Autodesk Fusion 360 part; units mm, degrees
note: some values were not read from the file. Set by a fixed rule: which sketch regions a step uses.
(part 3 of 7)
sketch "Sketch57" plane through (0, 116.2145, -31.1396) normal (0, 0.965926, -0.258819) x (-1, 0, 0)
  line L0 (-36.6, 185) -> (-48.311, 185)
  arc A0 (-49.911, 186.6) -> (-48.311, 185) centre (-48.311, 186.6) ccw
  line L1 (-49.911, 186.6) -> (-49.911, 195.348)
  arc A1 (-48.311, 196.948) -> (-49.911, 195.348) centre (-48.311, 195.348) ccw
  line L2 (-48.311, 196.948) -> (-36.6, 196.948)
  arc A2 (-35, 195.348) -> (-36.6, 196.948) centre (-36.6, 195.348) ccw
  line L3 (-35, 195.348) -> (-35, 186.6)
  arc A3 (-36.6, 185) -> (-35, 186.6) centre (-36.6, 186.6) ccw
  line L4 (-55, 195.348) -> (-55, 186.6)
  arc A4 (-56.6, 185) -> (-55, 186.6) centre (-56.6, 186.6) ccw
  line L5 (-56.6, 185) -> (-68.3957, 185)
  arc A5 (-69.9957, 186.6) -> (-68.3957, 185) centre (-68.3957, 186.6) ccw
  line L6 (-69.9957, 186.6) -> (-69.9957, 195.348)
  arc A6 (-68.3957, 196.948) -> (-69.9957, 195.348) centre (-68.3957, 195.348) ccw
  line L7 (-68.3957, 196.948) -> (-56.6, 196.948)
  arc A7 (-55, 195.348) -> (-56.6, 196.948) centre (-56.6, 195.348) ccw
  line L8 (-35, 204.6984) -> (-35, 201.6)
  arc A8 (-36.6, 200) -> (-35, 201.6) centre (-36.6, 201.6) ccw
  line L9 (-36.6, 200) -> (-48.311, 200)
  arc A9 (-49.911, 201.6) -> (-48.311, 200) centre (-48.311, 201.6) ccw
  line L10 (-49.911, 201.6) -> (-49.911, 204.6984)
  arc A10 (-48.311, 206.2984) -> (-49.911, 204.6984) centre (-48.311, 204.6984) ccw
  line L11 (-48.311, 206.2984) -> (-36.6, 206.2984)
  arc A11 (-35, 204.6984) -> (-36.6, 206.2984) centre (-36.6, 204.6984) ccw
  line L12 (-55, 204.5671) -> (-55, 201.6)
  arc A12 (-56.6, 200) -> (-55, 201.6) centre (-56.6, 201.6) ccw
  line L13 (-56.6, 200) -> (-68.7895, 200)
  arc A13 (-70.3895, 201.6) -> (-68.7895, 200) centre (-68.7895, 201.6) ccw
  line L14 (-70.3895, 201.6) -> (-70.3895, 204.5671)
  arc A14 (-68.7895, 206.1671) -> (-70.3895, 204.5671) centre (-68.7895, 204.5671) ccw
  line L15 (-68.7895, 206.1671) -> (-56.6, 206.1671)
  arc A15 (-55, 204.5671) -> (-56.6, 206.1671) centre (-56.6, 204.5671) ccw
  line L16 (25, 185) -> (0, 175)
  line L17 (0, 175) -> (0, 180.1897)
  line L18 (0, 180.1897) -> (25, 190.1897)
  line L19 (25, 190.1897) -> (25, 185)
  line L20 (-5, 190) -> (-5, 184.9041)
  line L21 (-5, 184.9041) -> (-30, 189.9041)
  line L22 (-30, 189.9041) -> (-30, 195)
  line L23 (-30, 195) -> (-5, 190)
  line L24 (-30, 150) -> (-30, 155)
  line L25 (-30, 155) -> (-5, 150)
  line L26 (-5, 150) -> (-5, 145)
  line L27 (-5, 145) -> (-30, 150)
  line L28 (-30, 160) -> (-30, 165.149)
  line L29 (-30, 165.149) -> (-5, 160.149)
  line L30 (-5, 160.149) -> (-5, 155)
  line L31 (-5, 155) -> (-30, 160)
  line L32 (-30, 200) -> (-30, 205)
  line L33 (-30, 205) -> (-5, 200)
  line L34 (-5, 200) -> (-5, 195)
  line L35 (-5, 195) -> (-30, 200)
  line L36 (25, 180.1705) -> (25, 175)
  line L37 (25, 175) -> (0, 165)
  line L38 (0, 165) -> (0, 170)
  line L39 (0, 170) -> (25, 180.1705)
  line L40 (25, 155) -> (0, 145)
  line L41 (0, 145) -> (0, 150)
  line L42 (0, 150) -> (25, 160)
  line L43 (25, 160) -> (25, 155)
  line L44 (25, 195) -> (0, 185)
  line L45 (0, 185) -> (0, 190)
  line L46 (0, 190) -> (25, 200)
  line L47 (25, 200) -> (25, 195)
  line L48 (-30, 180) -> (-30, 184.9041)
  line L49 (-30, 184.9041) -> (-5, 180)
  line L50 (-5, 180) -> (-5, 175)
  line L51 (-5, 175) -> (-30, 180)
  line L52 (-30, 170) -> (-30, 175)
  line L53 (-30, 175) -> (-5, 170)
  line L54 (-5, 170) -> (-5, 165)
  line L55 (-5, 165) -> (-30, 170)
  line L56 (25, 205) -> (0, 195)
  line L57 (0, 195) -> (0, 200)
  line L58 (0, 200) -> (25, 210)
  line L59 (25, 210) -> (25, 205)
  line L60 (25, 165) -> (0, 155)
  line L61 (0, 155) -> (0, 160)
  line L62 (0, 160) -> (25, 170)
  line L63 (25, 170) -> (25, 165)
  line L64 (-109.8689, 117.075) -> (-111.5449, 117.075)
  arc A16 (-116.5449, 122.075) -> (-111.5449, 117.075) centre (-111.5449, 122.075) ccw
  line L65 (-116.5449, 122.075) -> (-116.5449, 197.0502)
  arc A17 (-111.5449, 202.0502) -> (-116.5449, 197.0502) centre (-111.5449, 197.0502) ccw
  line L66 (-111.5449, 202.0502) -> (-109.8689, 202.0502)
  arc A18 (-104.8689, 197.0502) -> (-109.8689, 202.0502) centre (-109.8689, 197.0502) ccw
  line L67 (-104.8689, 197.0502) -> (-104.8689, 122.075)
  arc A19 (-109.8689, 117.075) -> (-104.8689, 122.075) centre (-109.8689, 122.075) ccw
  line L68 (-35, 125) -> (-35, 117.5)
  arc A20 (-37.5, 115) -> (-35, 117.5) centre (-37.5, 117.5) ccw
  line L69 (-37.5, 115) -> (-65, 115)
  arc A21 (-70, 120) -> (-65, 115) centre (-65, 120) ccw
  line L70 (-70, 120) -> (-70, 125)
  arc A22 (-65, 130) -> (-70, 125) centre (-65, 125) ccw
  line L71 (-65, 130) -> (-40, 130)
  arc A23 (-35, 125) -> (-40, 130) centre (-40, 125) ccw
  line L72 (-95.5983, 117.0948) -> (-95.6526, 117.0948)
  arc A24 (-100.6526, 122.0948) -> (-95.6526, 117.0948) centre (-95.6526, 122.0948) ccw
  line L73 (-100.6526, 122.0948) -> (-100.6526, 154.3733)
  line L74 (-100.6526, 154.3733) -> (-90.5983, 154.3733)
  line L75 (-90.5983, 154.3733) -> (-90.5983, 122.0948)
  arc A25 (-95.5983, 117.0948) -> (-90.5983, 122.0948) centre (-95.5983, 122.0948) ccw
  arc A26 (-90.5983, 197.0502) -> (-95.5983, 202.0502) centre (-95.5983, 197.0502) ccw
  line L76 (-90.5983, 197.0502) -> (-90.5983, 159.5626)
  line L77 (-90.5983, 159.5626) -> (-100.6526, 159.5626)
  line L78 (-100.6526, 159.5626) -> (-100.6526, 197.0502)
  arc A27 (-95.6526, 202.0502) -> (-100.6526, 197.0502) centre (-95.6526, 197.0502) ccw
  line L79 (-95.6526, 202.0502) -> (-95.5983, 202.0502)
  line L80 (-37.5, 135) -> (-67.5, 135)
  arc A28 (-70, 137.5) -> (-67.5, 135) centre (-67.5, 137.5) ccw
  line L81 (-70, 137.5) -> (-70, 142.5)
  arc A29 (-67.5, 145) -> (-70, 142.5) centre (-67.5, 142.5) ccw
  line L82 (-67.5, 145) -> (-37.5, 145)
  arc A30 (-35, 142.5) -> (-37.5, 145) centre (-37.5, 142.5) ccw
  line L83 (-35, 142.5) -> (-35, 137.5)
  arc A31 (-37.5, 135) -> (-35, 137.5) centre (-37.5, 137.5) ccw
  arc A32 (-84.2974, 121.8844) -> (-80.3534, 116.9972) centre (-79.2974, 121.8844) ccw
  line L84 (-84.2974, 121.8844) -> (-84.2974, 171.0352)
  line L85 (-84.2974, 171.0352) -> (-76.4093, 171.0352)
  line L86 (-76.4093, 171.0352) -> (-76.4093, 121.8844)
  arc A33 (-80.3534, 116.9972) -> (-76.4093, 121.8844) centre (-81.4093, 121.8844) ccw
  arc A34 (-76.4093, 196.948) -> (-80.3534, 201.8353) centre (-81.4093, 196.948) ccw
  line L87 (-76.4093, 196.948) -> (-76.4093, 176.5782)
  line L88 (-76.4093, 176.5782) -> (-84.2974, 176.5782)
  line L89 (-84.2974, 176.5782) -> (-84.2974, 196.948)
  arc A35 (-80.3534, 201.8353) -> (-84.2974, 196.948) centre (-79.2974, 196.948) ccw
  line L90 (-120, 85) -> (-120, 100)
  arc A36 (-110, 110) -> (-120, 100) centre (-110, 100) ccw
  line L91 (-110, 110) -> (-61.6636, 110)
  arc A37 (-51.6636, 100) -> (-61.6636, 110) centre (-61.6636, 100) ccw
  line L92 (-51.6636, 100) -> (-51.6636, 85)
  arc A38 (-61.6636, 75) -> (-51.6636, 85) centre (-61.6636, 85) ccw
  line L93 (-61.6636, 75) -> (-110, 75)
  arc A39 (-120, 85) -> (-110, 75) centre (-110, 85) ccw
  line L94 (-45.44, 85) -> (-45.44, 100)
  arc A40 (-35.44, 110) -> (-45.44, 100) centre (-35.44, 100) ccw
  line L95 (-35.44, 110) -> (-20, 110)
  arc A41 (-10, 100) -> (-20, 110) centre (-20, 100) ccw
  line L96 (-10, 100) -> (-10, 85)
  arc A42 (-20, 75) -> (-10, 85) centre (-20, 85) ccw
  line L97 (-20, 75) -> (-35.44, 75)
  arc A43 (-45.44, 85) -> (-35.44, 75) centre (-35.44, 85) ccw
  line L98 (22.9316, 100) -> (22.9316, 85)
  arc A44 (12.9316, 75) -> (22.9316, 85) centre (12.9316, 85) ccw
  line L99 (12.9316, 75) -> (7.9281, 75)
  arc A45 (-2.0719, 85) -> (7.9281, 75) centre (7.9281, 85) ccw
  line L100 (-2.0719, 85) -> (-2.0719, 100)
  arc A46 (7.9281, 110) -> (-2.0719, 100) centre (7.9281, 100) ccw
  line L101 (7.9281, 110) -> (12.9316, 110)
  arc A47 (22.9316, 100) -> (12.9316, 110) centre (12.9316, 100) ccw
  line L102 (-40, 30) -> (-110, 30)
  arc A48 (-120, 40) -> (-110, 30) centre (-110, 40) ccw
  line L103 (-120, 40) -> (-120, 60)
  arc A49 (-110, 70) -> (-120, 60) centre (-110, 60) ccw
  line L104 (-110, 70) -> (-40, 70)
  arc A50 (-30, 60) -> (-40, 70) centre (-40, 60) ccw
  line L105 (-30, 60) -> (-30, 40)
  arc A51 (-40, 30) -> (-30, 40) centre (-40, 40) ccw
  line L106 (-10, 70) -> (10, 70)
  arc A52 (20, 60) -> (10, 70) centre (10, 60) ccw
  line L107 (20, 60) -> (20, 40)
  arc A53 (10, 30) -> (20, 40) centre (10, 40) ccw
  line L108 (10, 30) -> (-10, 30)
  arc A54 (-20, 40) -> (-10, 30) centre (-10, 40) ccw
  line L109 (-20, 40) -> (-20, 60)
  arc A55 (-10, 70) -> (-20, 60) centre (-10, 60) ccw
  ellipse E0 centre (22.741, -39.3535) end of major axis (22.741, -46.5838) minor radius 7 (22.741, -46.5838) -> (29.741, -39.3535) ccw
  line L110 (29.741, -39.3535) -> (29.741, 209.5755)
  ellipse E1 centre (22.741, 209.5755) end of major axis (22.741, 216.8058) minor radius 7 (29.741, 209.5755) -> (22.741, 216.8058) ccw
  line L111 (22.741, 216.8058) -> (-123.259, 216.8058)
  ellipse E2 centre (-123.259, 209.5755) end of major axis (-123.259, 216.8058) minor radius 7 (-123.259, 216.8058) -> (-130.259, 209.5755) ccw
  line L112 (-130.259, 209.5755) -> (-130.259, -39.3535)
  ellipse E3 centre (-123.259, -39.3535) end of major axis (-123.259, -46.5838) minor radius 7 (-130.259, -39.3535) -> (-123.259, -46.5838) ccw
  line L113 (-123.259, -46.5838) -> (22.741, -46.5838)
  line L114 (-35.9419, 179.9959) -> (-35.9419, 150.9959)
  line L115 (-35.9419, 150.9959) -> (-72.9419, 150.9959)
  line L116 (-72.9419, 150.9959) -> (-72.9419, 179.9959)
  line L117 (-72.9419, 179.9959) -> (-35.9419, 179.9959)
  circle A56 centre (-57, 13) radius 1.5
  dimension "d224" = 3
  measures "d224" diameter of A56
sketch "Sketch58" plane through (0, 0, 0) normal (0, 1, 0) x (1, 0, 0)
sketch "Sketch1 (2)" plane through (0, 0, 0) normal (0, 1, 0) x (1, 0, 0) in component "axe"
  line L0 (-180, -19.5879) -> (-227.1834, -19.5879)
  line L1 (-227.1834, -19.5879) -> (-227.1834, -2.995)
  line L2 (-227.1834, -2.995) -> (-170, -2.995)
  line L3 (-170, -2.995) -> (-170, -9.5879)
  line L4 (-189.6546, -2.995) -> (-208.419, -2.995)
  line L5 (-208.419, -2.995) -> (-208.419, 108.2304)
  line L6 (-208.419, 108.2304) -> (-189.6546, 108.2304)
  line L7 (-189.6546, 108.2304) -> (-189.6546, -2.995)
  arc A0 (-180, -19.5879) -> (-170, -9.5879) centre (-180, -9.5879) ccw
  dimension "d328" = 10
  dimension "d329" = 127.8184
  constraint horizontal L0
  constraint vertical L1
  constraint horizontal L2
  constraint vertical L3
  constraint horizontal L4
  constraint vertical L5
  constraint horizontal L6
  constraint vertical L7
  constraint coincident L2 L4.start
  constraint tangent L0 A0
  constraint tangent L3 A0
  measures "d328" radius of A0
  measures "d329" distance of L0 L6
extrude "Extrude1" add sketch "Sketch1 (2)" along normal blind 10 in component "axe"
shell "Shell1" thickness 1 removed faces 1 at (-202.1642, 3.3333, -108.2304) in component "axe"
move_body "Move1" bodies 1 to x (1, 0, 0) y (0, -1, 0) z (0, 0, -1) at (237.3583, 174.6092, -54.5958) in component "axe"
move_body "Move2" bodies 1 to x (0, 1, 0) y (-1, 0, 0) z (0, 0, 1) at (222.3129, 121.9056, 15) in component "axe"
move_body "Move3" bodies 1 to x (1, 0, 0) y (0, 0.258819, 0.965926) z (0, -0.965926, 0.258819) at (3.5, 142.9141, -113.2543) in component "axe"
move_body "Move4" bodies 1 to x (1, 0, 0) y (0, 1, 0) z (0, 0, 1) at (170, 47.007, -22.6429) in component "axe"
sketch "Sketch60" plane through (-29.741, 0, 0) normal (-1, 0, 0) x (0, 0, 1)
  line L0 (4.8558, 108) -> (45, 108)
  line L1 (45, 108) -> (45, 101.218)
  line L2 (45, 101.218) -> (4.8558, 101.218)
  line L3 (4.8558, 101.218) -> (4.8558, 108)
  line L4 (-69.1521, 106.0291) -> (-69.1009, 100.1665)
  line L5 (-69.1009, 100.1665) -> (171.8899, 102.2696)
  line L6 (171.8899, 102.2696) -> (171.2948, 170.4566)
  line L7 (171.2948, 170.4566) -> (-69.1521, 106.0291)
  line L8 (103.7389, 125) -> (70, 125)
  line L9 (65, 120) -> (65, 115.8193)
  line L10 (70, 110.8193) -> (103.7389, 110.8193)
  line L11 (108.7389, 115.8193) -> (108.7389, 120)
  arc A0 (70, 125) -> (65, 120) centre (70, 120) ccw
  arc A1 (65, 115.8193) -> (70, 110.8193) centre (70, 115.8193) ccw
  arc A2 (108.7389, 120) -> (103.7389, 125) centre (103.7389, 120) ccw
  arc A3 (103.7389, 110.8193) -> (108.7389, 115.8193) centre (103.7389, 115.8193) ccw
  dimension "d243" = 5
  dimension "d244" = 5
  constraint horizontal L8
  constraint vertical L9
  constraint horizontal L10
  constraint vertical L11
  constraint tangent L8 A0
  constraint tangent L9 A0
  constraint tangent L9 A1
  constraint tangent L10 A1
  constraint equal A0 A1
  constraint tangent L8 A2
  constraint tangent L11 A2
  constraint tangent L10 A3
  constraint tangent L11 A3
  constraint equal A2 A3
  measures "d243" radius of A0
  measures "d244" radius of A2
sketch "Sketch61" plane through (130.259, 0, 0) normal (1, 0, 0) x (0, 0, -1)
  line L0 (-45, 101.218) -> (-45, 110)
  line L1 (-45, 110) -> (-6.7003, 110)
  line L2 (-6.7003, 110) -> (-6.7003, 101.218)
  line L3 (-6.7003, 101.218) -> (-45, 101.218)
  line L4 (69.1009, 100.1665) -> (69.1521, 106.0291)
  line L5 (69.1521, 106.0291) -> (-171.2948, 170.4566)
  line L6 (-171.2948, 170.4566) -> (-171.8899, 102.2696)
  line L7 (-171.8899, 102.2696) -> (69.1009, 100.1665)
  line L8 (-108.8645, 127.2667) -> (-70.0825, 127.2667)
  line L9 (-66.3825, 123.5667) -> (-66.3825, 116.3937)
  line L10 (-70.0825, 112.6937) -> (-108.8645, 112.6937)
  line L11 (-112.5645, 116.3937) -> (-112.5645, 123.5667)
  arc A0 (-66.3825, 123.5667) -> (-70.0825, 127.2667) centre (-70.0825, 123.5667) ccw
  arc A1 (-70.0825, 112.6937) -> (-66.3825, 116.3937) centre (-70.0825, 116.3937) ccw
  arc A2 (-112.5645, 116.3937) -> (-108.8645, 112.6937) centre (-108.8645, 116.3937) ccw
  arc A3 (-108.8645, 127.2667) -> (-112.5645, 123.5667) centre (-108.8645, 123.5667) ccw
  dimension "d247" = 3.7
  constraint horizontal L8
  constraint horizontal L10
  constraint vertical L11
  constraint tangent L8 A0
  constraint tangent L9 A0
  constraint tangent L9 A1
  constraint tangent L10 A1
  constraint equal A0 A1
  constraint tangent L10 A2
  constraint tangent L11 A2
  constraint equal A0 A2
  constraint tangent L8 A3
  constraint tangent L11 A3
  constraint equal A0 A3
  measures "d247" radius of A0
sketch "Sketch62" plane through (-26.741, 0, 0) normal (1, 0, 0) x (0, 0, -1)
  line L0 (-175.8897, 102.3045) -> (73.1008, 100.1316)
  line L1 (73.1008, 100.1316) -> (73.1159, 101.8612)
  line L2 (73.1159, 101.8612) -> (-175.3127, 168.4274)
  line L3 (-175.3127, 168.4274) -> (-175.8897, 102.3045)
  line L4 (-101.4003, 140.9215) -> (-77.5652, 140.9215)
  line L5 (-77.5652, 140.9215) -> (-77.5652, 128.7199)
  line L6 (-77.5652, 128.7199) -> (-101.4003, 128.7199)
  line L7 (-101.4003, 128.7199) -> (-101.4003, 140.9215)
  constraint horizontal L4
  constraint vertical L5
  constraint horizontal L6
  constraint vertical L7
move_body "Move5" bodies 1 to x (1, 0, 0) y (0, 1, 0) z (0, 0, 1) at (-87, -50.9421, 56.6747) in component "axe"
sketch "Sketch64" plane through (0, 115.0071, -30.8161) normal (0, 0.965926, -0.258819) x (-1, 0, 0)
  arc A0 (-110, 110) -> (-120, 100) centre (-110, 100) ccw
  line L0 (-120, 100) -> (-120, 85)
  arc A1 (-120, 85) -> (-110, 75) centre (-110, 85) ccw
  line L1 (-110, 75) -> (-61.6636, 75)
  arc A2 (-61.6636, 75) -> (-51.6636, 85) centre (-61.6636, 85) ccw
  line L2 (-51.6636, 85) -> (-51.6636, 100)
  arc A3 (-51.6636, 100) -> (-61.6636, 110) centre (-61.6636, 100) ccw
  line L3 (-61.6636, 110) -> (-110, 110)
sketch "Sketch65" plane through (0, 115.0071, -30.8161) normal (0, 0.965926, -0.258819) x (-1, 0, 0)
  line L0 (-110, 110) -> (-82.9094, 110)
  line L1 (-82.9094, 110) -> (-82.9094, 88.2587)
  line L2 (-82.9094, 88.2587) -> (-110, 88.2587)
  line L3 (-110, 88.2587) -> (-110, 110)
  line L4 (-65, 80) -> (-96.4547, 80)
  line L5 (-96.4547, 80) -> (-96.4547, 101.0146)
  line L6 (-96.4547, 101.0146) -> (-65, 101.0146)
  line L7 (-65, 101.0146) -> (-65, 80)
  line L8 (-52.1358, 86.6643) -> (-76.8504, 86.6643)
  line L9 (-76.8504, 86.6643) -> (-76.8504, 104.6819)
  line L10 (-76.8504, 104.6819) -> (-52.1358, 104.6819)
  line L11 (-52.1358, 104.6819) -> (-52.1358, 86.6643)
  line L12 (-102.5797, 95.6731) -> (-115, 95.6731)
  line L13 (-115, 95.6731) -> (-115, 80)
  line L14 (-115, 80) -> (-102.5797, 80)
  line L15 (-102.5797, 80) -> (-102.5797, 95.6731)
  constraint horizontal L0
  constraint vertical L1
  constraint horizontal L2
  constraint vertical L3
  constraint horizontal L4
  constraint vertical L5
  constraint horizontal L6
  constraint vertical L7
  constraint horizontal L8
  constraint vertical L9
  constraint horizontal L10
  constraint vertical L11
  constraint horizontal L12
  constraint vertical L13
  constraint horizontal L14
  constraint vertical L15
sketch "Sketch66" plane through (0, 115.0071, -30.8161) normal (0, 0.965926, -0.258819) x (-1, 0, 0)
  line L0 (-110, 75) -> (-90, 75)
  line L1 (-90, 75) -> (-90, 95)
  line L2 (-90, 95) -> (-110, 95)
  line L3 (-110, 95) -> (-110, 75)
  line L4 (-60, 80) -> (-81.2122, 80)
  line L5 (-81.2122, 80) -> (-81.2122, 98.5014)
  line L6 (-81.2122, 98.5014) -> (-60, 98.5014)
  line L7 (-60, 98.5014) -> (-60, 80)
  constraint horizontal L0
  constraint vertical L1
  constraint horizontal L2
  constraint vertical L3
  constraint horizontal L4
  constraint vertical L5
  constraint horizontal L6
  constraint vertical L7
sketch "Sketch67" plane through (0, 115.973, -31.0749) normal (0, 0.965926, -0.258819) x (-1, 0, 0)
  line L0 (-60, 98.5014) -> (-81.2122, 98.5014)
  line L1 (-81.2122, 98.5014) -> (-81.2122, 80)
  line L2 (-81.2122, 80) -> (-60, 80)
  line L3 (-60, 80) -> (-60, 98.5014)
  circle A0 centre (-63, 96) radius 1.5
  circle A1 centre (-78, 96) radius 1.5
  circle A2 centre (-93, 92) radius 1.5
  circle A3 centre (-107, 92) radius 1.5
  dimension "d262" = 3
  dimension "d263" = 3
  dimension "d264" = 3
  dimension "d265" = 3
  measures "d262" diameter of A0
  measures "d263" diameter of A1
  measures "d264" diameter of A2
  measures "d265" diameter of A3
move_body "Move6" bodies 1 to x (1, 0, 0) y (0, 1, 0) z (0, 0, 1) at (138.1861, 0.7755, 2.894) in component "axe"
sketch "Sketch70" plane through (0, 116.2145, -31.1396) normal (0, 0.965926, -0.258819) x (-1, 0, 0)
  line L0 (-36.6, 185) -> (-48.311, 185)
  arc A0 (-49.911, 186.6) -> (-48.311, 185) centre (-48.311, 186.6) ccw
  line L1 (-49.911, 186.6) -> (-49.911, 195.348)
  arc A1 (-48.311, 196.948) -> (-49.911, 195.348) centre (-48.311, 195.348) ccw
  line L2 (-48.311, 196.948) -> (-36.6, 196.948)
  arc A2 (-35, 195.348) -> (-36.6, 196.948) centre (-36.6, 195.348) ccw
  line L3 (-35, 195.348) -> (-35, 186.6)
  arc A3 (-36.6, 185) -> (-35, 186.6) centre (-36.6, 186.6) ccw
  line L4 (-55, 195.348) -> (-55, 186.6)
  arc A4 (-56.6, 185) -> (-55, 186.6) centre (-56.6, 186.6) ccw
  line L5 (-56.6, 185) -> (-68.3957, 185)
  arc A5 (-69.9957, 186.6) -> (-68.3957, 185) centre (-68.3957, 186.6) ccw
  line L6 (-69.9957, 186.6) -> (-69.9957, 195.348)
  arc A6 (-68.3957, 196.948) -> (-69.9957, 195.348) centre (-68.3957, 195.348) ccw
  line L7 (-68.3957, 196.948) -> (-56.6, 196.948)
  arc A7 (-55, 195.348) -> (-56.6, 196.948) centre (-56.6, 195.348) ccw
  line L8 (-35, 204.6984) -> (-35, 201.6)
  arc A8 (-36.6, 200) -> (-35, 201.6) centre (-36.6, 201.6) ccw
  line L9 (-36.6, 200) -> (-48.311, 200)
  arc A9 (-49.911, 201.6) -> (-48.311, 200) centre (-48.311, 201.6) ccw
  line L10 (-49.911, 201.6) -> (-49.911, 204.6984)
  arc A10 (-48.311, 206.2984) -> (-49.911, 204.6984) centre (-48.311, 204.6984) ccw
  line L11 (-48.311, 206.2984) -> (-36.6, 206.2984)
  arc A11 (-35, 204.6984) -> (-36.6, 206.2984) centre (-36.6, 204.6984) ccw
  line L12 (-55, 204.5671) -> (-55, 201.6)
  arc A12 (-56.6, 200) -> (-55, 201.6) centre (-56.6, 201.6) ccw
  line L13 (-56.6, 200) -> (-68.7895, 200)
  arc A13 (-70.3895, 201.6) -> (-68.7895, 200) centre (-68.7895, 201.6) ccw
  line L14 (-70.3895, 201.6) -> (-70.3895, 204.5671)
  arc A14 (-68.7895, 206.1671) -> (-70.3895, 204.5671) centre (-68.7895, 204.5671) ccw
  line L15 (-68.7895, 206.1671) -> (-56.6, 206.1671)
  arc A15 (-55, 204.5671) -> (-56.6, 206.1671) centre (-56.6, 204.5671) ccw
  line L16 (25, 185) -> (0, 175)
  line L17 (0, 175) -> (0, 180.1897)
  line L18 (0, 180.1897) -> (25, 190.1897)
  line L19 (25, 190.1897) -> (25, 185)
  line L20 (-5, 190) -> (-5, 184.9041)
  line L21 (-5, 184.9041) -> (-30, 189.9041)
  line L22 (-30, 189.9041) -> (-30, 195)
  line L23 (-30, 195) -> (-5, 190)
  line L24 (-30, 150) -> (-30, 155)
  line L25 (-30, 155) -> (-5, 150)
  line L26 (-5, 150) -> (-5, 145)
  line L27 (-5, 145) -> (-30, 150)
  line L28 (-30, 160) -> (-30, 165.149)
  line L29 (-30, 165.149) -> (-5, 160.149)
  line L30 (-5, 160.149) -> (-5, 155)
  line L31 (-5, 155) -> (-30, 160)
  line L32 (-30, 200) -> (-30, 205)
  line L33 (-30, 205) -> (-5, 200)
  line L34 (-5, 200) -> (-5, 195)
  line L35 (-5, 195) -> (-30, 200)
  line L36 (25, 180.1705) -> (25, 175)
  line L37 (25, 175) -> (0, 165)
  line L38 (0, 165) -> (0, 170)
  line L39 (0, 170) -> (25, 180.1705)
  line L40 (25, 155) -> (0, 145)
  line L41 (0, 145) -> (0, 150)
  line L42 (0, 150) -> (25, 160)
  line L43 (25, 160) -> (25, 155)
  line L44 (25, 195) -> (0, 185)
  line L45 (0, 185) -> (0, 190)
  line L46 (0, 190) -> (25, 200)
  line L47 (25, 200) -> (25, 195)
  line L48 (-30, 180) -> (-30, 184.9041)
  line L49 (-30, 184.9041) -> (-5, 180)
  line L50 (-5, 180) -> (-5, 175)
  line L51 (-5, 175) -> (-30, 180)
  line L52 (-30, 170) -> (-30, 175)
  line L53 (-30, 175) -> (-5, 170)
  line L54 (-5, 170) -> (-5, 165)
  line L55 (-5, 165) -> (-30, 170)
  line L56 (25, 205) -> (0, 195)
  line L57 (0, 195) -> (0, 200)
  line L58 (0, 200) -> (25, 210)
  line L59 (25, 210) -> (25, 205)
  line L60 (25, 165) -> (0, 155)
  line L61 (0, 155) -> (0, 160)
  line L62 (0, 160) -> (25, 170)
  line L63 (25, 170) -> (25, 165)
  line L64 (-109.8689, 117.075) -> (-111.5449, 117.075)
  arc A16 (-116.5449, 122.075) -> (-111.5449, 117.075) centre (-111.5449, 122.075) ccw
  line L65 (-116.5449, 122.075) -> (-116.5449, 197.0502)
  arc A17 (-111.5449, 202.0502) -> (-116.5449, 197.0502) centre (-111.5449, 197.0502) ccw
  line L66 (-111.5449, 202.0502) -> (-109.8689, 202.0502)
  arc A18 (-104.8689, 197.0502) -> (-109.8689, 202.0502) centre (-109.8689, 197.0502) ccw
  line L67 (-104.8689, 197.0502) -> (-104.8689, 122.075)
  arc A19 (-109.8689, 117.075) -> (-104.8689, 122.075) centre (-109.8689, 122.075) ccw
  line L68 (-35, 125) -> (-35, 117.5)
  arc A20 (-37.5, 115) -> (-35, 117.5) centre (-37.5, 117.5) ccw
  line L69 (-37.5, 115) -> (-65, 115)
  arc A21 (-70, 120) -> (-65, 115) centre (-65, 120) ccw
  line L70 (-70, 120) -> (-70, 125)
  arc A22 (-65, 130) -> (-70, 125) centre (-65, 125) ccw
  line L71 (-65, 130) -> (-40, 130)
  arc A23 (-35, 125) -> (-40, 130) centre (-40, 125) ccw
  line L72 (-95.5983, 117.0948) -> (-95.6526, 117.0948)
  arc A24 (-100.6526, 122.0948) -> (-95.6526, 117.0948) centre (-95.6526, 122.0948) ccw
  line L73 (-100.6526, 122.0948) -> (-100.6526, 154.3733)
  line L74 (-100.6526, 154.3733) -> (-90.5983, 154.3733)
  line L75 (-90.5983, 154.3733) -> (-90.5983, 122.0948)
  arc A25 (-95.5983, 117.0948) -> (-90.5983, 122.0948) centre (-95.5983, 122.0948) ccw
  arc A26 (-90.5983, 197.0502) -> (-95.5983, 202.0502) centre (-95.5983, 197.0502) ccw
  line L76 (-90.5983, 197.0502) -> (-90.5983, 159.5626)
  line L77 (-90.5983, 159.5626) -> (-100.6526, 159.5626)
  line L78 (-100.6526, 159.5626) -> (-100.6526, 197.0502)
  arc A27 (-95.6526, 202.0502) -> (-100.6526, 197.0502) centre (-95.6526, 197.0502) ccw
  line L79 (-95.6526, 202.0502) -> (-95.5983, 202.0502)
  line L80 (-37.5, 135) -> (-67.5, 135)
  arc A28 (-70, 137.5) -> (-67.5, 135) centre (-67.5, 137.5) ccw
  line L81 (-70, 137.5) -> (-70, 142.5)
  arc A29 (-67.5, 145) -> (-70, 142.5) centre (-67.5, 142.5) ccw
  line L82 (-67.5, 145) -> (-37.5, 145)
  arc A30 (-35, 142.5) -> (-37.5, 145) centre (-37.5, 142.5) ccw
  line L83 (-35, 142.5) -> (-35, 137.5)
  arc A31 (-37.5, 135) -> (-35, 137.5) centre (-37.5, 137.5) ccw
  arc A32 (-84.2974, 121.8844) -> (-80.3534, 116.9972) centre (-79.2974, 121.8844) ccw
  line L84 (-84.2974, 121.8844) -> (-84.2974, 171.0352)
  line L85 (-84.2974, 171.0352) -> (-76.4093, 171.0352)
  line L86 (-76.4093, 171.0352) -> (-76.4093, 121.8844)
  arc A33 (-80.3534, 116.9972) -> (-76.4093, 121.8844) centre (-81.4093, 121.8844) ccw
  arc A34 (-76.4093, 196.948) -> (-80.3534, 201.8353) centre (-81.4093, 196.948) ccw
  line L87 (-76.4093, 196.948) -> (-76.4093, 176.5782)
  line L88 (-76.4093, 176.5782) -> (-84.2974, 176.5782)
  line L89 (-84.2974, 176.5782) -> (-84.2974, 196.948)
  arc A35 (-80.3534, 201.8353) -> (-84.2974, 196.948) centre (-79.2974, 196.948) ccw
  line L90 (-120, 85) -> (-120, 100)
  arc A36 (-110, 110) -> (-120, 100) centre (-110, 100) ccw
  line L91 (-110, 110) -> (-61.6636, 110)
  arc A37 (-51.6636, 100) -> (-61.6636, 110) centre (-61.6636, 100) ccw
  line L92 (-51.6636, 100) -> (-51.6636, 85)
  arc A38 (-61.6636, 75) -> (-51.6636, 85) centre (-61.6636, 85) ccw
  line L93 (-61.6636, 75) -> (-110, 75)
  arc A39 (-120, 85) -> (-110, 75) centre (-110, 85) ccw
  line L94 (-45.44, 85) -> (-45.44, 100)
  arc A40 (-35.44, 110) -> (-45.44, 100) centre (-35.44, 100) ccw
  line L95 (-35.44, 110) -> (-20, 110)
  arc A41 (-10, 100) -> (-20, 110) centre (-20, 100) ccw
  line L96 (-10, 100) -> (-10, 85)
  arc A42 (-20, 75) -> (-10, 85) centre (-20, 85) ccw
  line L97 (-20, 75) -> (-35.44, 75)
  arc A43 (-45.44, 85) -> (-35.44, 75) centre (-35.44, 85) ccw
  line L98 (22.9316, 100) -> (22.9316, 85)
  arc A44 (12.9316, 75) -> (22.9316, 85) centre (12.9316, 85) ccw
  line L99 (12.9316, 75) -> (7.9281, 75)
  arc A45 (-2.0719, 85) -> (7.9281, 75) centre (7.9281, 85) ccw
  line L100 (-2.0719, 85) -> (-2.0719, 100)
  arc A46 (7.9281, 110) -> (-2.0719, 100) centre (7.9281, 100) ccw
  line L101 (7.9281, 110) -> (12.9316, 110)
  arc A47 (22.9316, 100) -> (12.9316, 110) centre (12.9316, 100) ccw
  line L102 (-40, 30) -> (-110, 30)
  arc A48 (-120, 40) -> (-110, 30) centre (-110, 40) ccw
  line L103 (-120, 40) -> (-120, 60)
  arc A49 (-110, 70) -> (-120, 60) centre (-110, 60) ccw
  line L104 (-110, 70) -> (-40, 70)
  arc A50 (-30, 60) -> (-40, 70) centre (-40, 60) ccw
  line L105 (-30, 60) -> (-30, 40)
  arc A51 (-40, 30) -> (-30, 40) centre (-40, 40) ccw
  line L106 (-10, 70) -> (10, 70)
  arc A52 (20, 60) -> (10, 70) centre (10, 60) ccw
  line L107 (20, 60) -> (20, 40)
  arc A53 (10, 30) -> (20, 40) centre (10, 40) ccw
  line L108 (10, 30) -> (-10, 30)
  arc A54 (-20, 40) -> (-10, 30) centre (-10, 40) ccw
  line L109 (-20, 40) -> (-20, 60)
  arc A55 (-10, 70) -> (-20, 60) centre (-10, 60) ccw
  ellipse E0 centre (22.741, -39.3535) end of major axis (22.741, -46.5838) minor radius 7 (22.741, -46.5838) -> (29.741, -39.3535) ccw
  line L110 (29.741, -39.3535) -> (29.741, 209.5755)
  ellipse E1 centre (22.741, 209.5755) end of major axis (22.741, 216.8058) minor radius 7 (29.741, 209.5755) -> (22.741, 216.8058) ccw
  line L111 (22.741, 216.8058) -> (-123.259, 216.8058)
  ellipse E2 centre (-123.259, 209.5755) end of major axis (-123.259, 216.8058) minor radius 7 (-123.259, 216.8058) -> (-130.259, 209.5755) ccw
  line L112 (-130.259, 209.5755) -> (-130.259, -39.3535)
  ellipse E3 centre (-123.259, -39.3535) end of major axis (-123.259, -46.5838) minor radius 7 (-130.259, -39.3535) -> (-123.259, -46.5838) ccw
  line L113 (-123.259, -46.5838) -> (22.741, -46.5838)
  line L114 (-35.9419, 179.9959) -> (-35.9419, 150.9959)
  line L115 (-35.9419, 150.9959) -> (-72.9419, 150.9959)
  line L116 (-72.9419, 150.9959) -> (-72.9419, 179.9959)
  line L117 (-72.9419, 179.9959) -> (-35.9419, 179.9959)
  line L118 (-60, 10) -> (-30.1991, 10)
  line L119 (-30.1991, 10) -> (-30.1991, -39.3535)
  line L120 (-30.1991, -39.3535) -> (-60, -39.3535)
  line L121 (-60, -39.3535) -> (-60, 10)
  constraint horizontal L118
  constraint vertical L119
  constraint horizontal L120
  constraint vertical L121
sketch "Sketch71" plane through (0, 116.2145, -31.1396) normal (0, 0.965926, -0.258819) x (-1, 0, 0)
  line L0 (-30.1991, -39.3535) -> (-60, -39.3535)
  line L1 (-36.6, 185) -> (-48.311, 185)
  arc A0 (-49.911, 186.6) -> (-48.311, 185) centre (-48.311, 186.6) ccw
  line L2 (-49.911, 186.6) -> (-49.911, 195.348)
  arc A1 (-48.311, 196.948) -> (-49.911, 195.348) centre (-48.311, 195.348) ccw
  line L3 (-48.311, 196.948) -> (-36.6, 196.948)
  arc A2 (-35, 195.348) -> (-36.6, 196.948) centre (-36.6, 195.348) ccw
  line L4 (-35, 195.348) -> (-35, 186.6)
  arc A3 (-36.6, 185) -> (-35, 186.6) centre (-36.6, 186.6) ccw
  line L5 (-55, 195.348) -> (-55, 186.6)
  arc A4 (-56.6, 185) -> (-55, 186.6) centre (-56.6, 186.6) ccw
  line L6 (-56.6, 185) -> (-68.3957, 185)
  arc A5 (-69.9957, 186.6) -> (-68.3957, 185) centre (-68.3957, 186.6) ccw
  line L7 (-69.9957, 186.6) -> (-69.9957, 195.348)
  arc A6 (-68.3957, 196.948) -> (-69.9957, 195.348) centre (-68.3957, 195.348) ccw
  line L8 (-68.3957, 196.948) -> (-56.6, 196.948)
  arc A7 (-55, 195.348) -> (-56.6, 196.948) centre (-56.6, 195.348) ccw
  line L9 (-35, 204.6984) -> (-35, 201.6)
  arc A8 (-36.6, 200) -> (-35, 201.6) centre (-36.6, 201.6) ccw
  line L10 (-36.6, 200) -> (-48.311, 200)
  arc A9 (-49.911, 201.6) -> (-48.311, 200) centre (-48.311, 201.6) ccw
  line L11 (-49.911, 201.6) -> (-49.911, 204.6984)
  arc A10 (-48.311, 206.2984) -> (-49.911, 204.6984) centre (-48.311, 204.6984) ccw
  line L12 (-48.311, 206.2984) -> (-36.6, 206.2984)
  arc A11 (-35, 204.6984) -> (-36.6, 206.2984) centre (-36.6, 204.6984) ccw
  line L13 (-55, 204.5671) -> (-55, 201.6)
  arc A12 (-56.6, 200) -> (-55, 201.6) centre (-56.6, 201.6) ccw
  line L14 (-56.6, 200) -> (-68.7895, 200)
  arc A13 (-70.3895, 201.6) -> (-68.7895, 200) centre (-68.7895, 201.6) ccw
  line L15 (-70.3895, 201.6) -> (-70.3895, 204.5671)
  arc A14 (-68.7895, 206.1671) -> (-70.3895, 204.5671) centre (-68.7895, 204.5671) ccw
  line L16 (-68.7895, 206.1671) -> (-56.6, 206.1671)
  arc A15 (-55, 204.5671) -> (-56.6, 206.1671) centre (-56.6, 204.5671) ccw
  line L17 (25, 185) -> (0, 175)
  line L18 (0, 175) -> (0, 180.1897)
  line L19 (0, 180.1897) -> (25, 190.1897)
  line L20 (25, 190.1897) -> (25, 185)
  line L21 (-5, 190) -> (-5, 184.9041)
  line L22 (-5, 184.9041) -> (-30, 189.9041)
  line L23 (-30, 189.9041) -> (-30, 195)
  line L24 (-30, 195) -> (-5, 190)
  line L25 (-30, 150) -> (-30, 155)
  line L26 (-30, 155) -> (-5, 150)
  line L27 (-5, 150) -> (-5, 145)
  line L28 (-5, 145) -> (-30, 150)
  line L29 (-30, 160) -> (-30, 165.149)
  line L30 (-30, 165.149) -> (-5, 160.149)
  line L31 (-5, 160.149) -> (-5, 155)
  line L32 (-5, 155) -> (-30, 160)
  line L33 (-30, 200) -> (-30, 205)
  line L34 (-30, 205) -> (-5, 200)
  line L35 (-5, 200) -> (-5, 195)
  line L36 (-5, 195) -> (-30, 200)
  line L37 (25, 180.1705) -> (25, 175)
  line L38 (25, 175) -> (0, 165)
  line L39 (0, 165) -> (0, 170)
  line L40 (0, 170) -> (25, 180.1705)
  line L41 (25, 155) -> (0, 145)
  line L42 (0, 145) -> (0, 150)
  line L43 (0, 150) -> (25, 160)
  line L44 (25, 160) -> (25, 155)
  line L45 (25, 195) -> (0, 185)
  line L46 (0, 185) -> (0, 190)
  line L47 (0, 190) -> (25, 200)
  line L48 (25, 200) -> (25, 195)
  line L49 (-30, 180) -> (-30, 184.9041)
  line L50 (-30, 184.9041) -> (-5, 180)
  line L51 (-5, 180) -> (-5, 175)
  line L52 (-5, 175) -> (-30, 180)
  line L53 (-30, 170) -> (-30, 175)
  line L54 (-30, 175) -> (-5, 170)
  line L55 (-5, 170) -> (-5, 165)
  line L56 (-5, 165) -> (-30, 170)
  line L57 (25, 205) -> (0, 195)
  line L58 (0, 195) -> (0, 200)
  line L59 (0, 200) -> (25, 210)
  line L60 (25, 210) -> (25, 205)
  line L61 (25, 165) -> (0, 155)
  line L62 (0, 155) -> (0, 160)
  line L63 (0, 160) -> (25, 170)
  line L64 (25, 170) -> (25, 165)
  line L65 (-109.8689, 117.075) -> (-111.5449, 117.075)
  arc A16 (-116.5449, 122.075) -> (-111.5449, 117.075) centre (-111.5449, 122.075) ccw
  line L66 (-116.5449, 122.075) -> (-116.5449, 197.0502)
  arc A17 (-111.5449, 202.0502) -> (-116.5449, 197.0502) centre (-111.5449, 197.0502) ccw
  line L67 (-111.5449, 202.0502) -> (-109.8689, 202.0502)
  arc A18 (-104.8689, 197.0502) -> (-109.8689, 202.0502) centre (-109.8689, 197.0502) ccw
  line L68 (-104.8689, 197.0502) -> (-104.8689, 122.075)
  arc A19 (-109.8689, 117.075) -> (-104.8689, 122.075) centre (-109.8689, 122.075) ccw
  line L69 (-35, 125) -> (-35, 117.5)
  arc A20 (-37.5, 115) -> (-35, 117.5) centre (-37.5, 117.5) ccw
  line L70 (-37.5, 115) -> (-65, 115)
  arc A21 (-70, 120) -> (-65, 115) centre (-65, 120) ccw
  line L71 (-70, 120) -> (-70, 125)
  arc A22 (-65, 130) -> (-70, 125) centre (-65, 125) ccw
  line L72 (-65, 130) -> (-40, 130)
  arc A23 (-35, 125) -> (-40, 130) centre (-40, 125) ccw
  line L73 (-95.5983, 117.0948) -> (-95.6526, 117.0948)
  arc A24 (-100.6526, 122.0948) -> (-95.6526, 117.0948) centre (-95.6526, 122.0948) ccw
  line L74 (-100.6526, 122.0948) -> (-100.6526, 154.3733)
  line L75 (-100.6526, 154.3733) -> (-90.5983, 154.3733)
  line L76 (-90.5983, 154.3733) -> (-90.5983, 122.0948)
  arc A25 (-95.5983, 117.0948) -> (-90.5983, 122.0948) centre (-95.5983, 122.0948) ccw
  arc A26 (-90.5983, 197.0502) -> (-95.5983, 202.0502) centre (-95.5983, 197.0502) ccw
  line L77 (-90.5983, 197.0502) -> (-90.5983, 159.5626)
  line L78 (-90.5983, 159.5626) -> (-100.6526, 159.5626)
  line L79 (-100.6526, 159.5626) -> (-100.6526, 197.0502)
  arc A27 (-95.6526, 202.0502) -> (-100.6526, 197.0502) centre (-95.6526, 197.0502) ccw
  line L80 (-95.6526, 202.0502) -> (-95.5983, 202.0502)
  line L81 (-37.5, 135) -> (-67.5, 135)
  arc A28 (-70, 137.5) -> (-67.5, 135) centre (-67.5, 137.5) ccw
  line L82 (-70, 137.5) -> (-70, 142.5)
  arc A29 (-67.5, 145) -> (-70, 142.5) centre (-67.5, 142.5) ccw
  line L83 (-67.5, 145) -> (-37.5, 145)
  arc A30 (-35, 142.5) -> (-37.5, 145) centre (-37.5, 142.5) ccw
  line L84 (-35, 142.5) -> (-35, 137.5)
  arc A31 (-37.5, 135) -> (-35, 137.5) centre (-37.5, 137.5) ccw
  arc A32 (-84.2974, 121.8844) -> (-80.3534, 116.9972) centre (-79.2974, 121.8844) ccw
  line L85 (-84.2974, 121.8844) -> (-84.2974, 171.0352)
  line L86 (-84.2974, 171.0352) -> (-76.4093, 171.0352)
  line L87 (-76.4093, 171.0352) -> (-76.4093, 121.8844)
  arc A33 (-80.3534, 116.9972) -> (-76.4093, 121.8844) centre (-81.4093, 121.8844) ccw
  arc A34 (-76.4093, 196.948) -> (-80.3534, 201.8353) centre (-81.4093, 196.948) ccw
  line L88 (-76.4093, 196.948) -> (-76.4093, 176.5782)
  line L89 (-76.4093, 176.5782) -> (-84.2974, 176.5782)
  line L90 (-84.2974, 176.5782) -> (-84.2974, 196.948)
  arc A35 (-80.3534, 201.8353) -> (-84.2974, 196.948) centre (-79.2974, 196.948) ccw
  line L91 (-120, 85) -> (-120, 100)
  arc A36 (-110, 110) -> (-120, 100) centre (-110, 100) ccw
  line L92 (-110, 110) -> (-61.6636, 110)
  arc A37 (-51.6636, 100) -> (-61.6636, 110) centre (-61.6636, 100) ccw
  line L93 (-51.6636, 100) -> (-51.6636, 85)
  arc A38 (-61.6636, 75) -> (-51.6636, 85) centre (-61.6636, 85) ccw
  line L94 (-61.6636, 75) -> (-110, 75)
  arc A39 (-120, 85) -> (-110, 75) centre (-110, 85) ccw
  line L95 (-45.44, 85) -> (-45.44, 100)
  arc A40 (-35.44, 110) -> (-45.44, 100) centre (-35.44, 100) ccw
  line L96 (-35.44, 110) -> (-20, 110)
  arc A41 (-10, 100) -> (-20, 110) centre (-20, 100) ccw
  line L97 (-10, 100) -> (-10, 85)
  arc A42 (-20, 75) -> (-10, 85) centre (-20, 85) ccw
  line L98 (-20, 75) -> (-35.44, 75)
  arc A43 (-45.44, 85) -> (-35.44, 75) centre (-35.44, 85) ccw
  line L99 (22.9316, 100) -> (22.9316, 85)
  arc A44 (12.9316, 75) -> (22.9316, 85) centre (12.9316, 85) ccw
  line L100 (12.9316, 75) -> (7.9281, 75)
  arc A45 (-2.0719, 85) -> (7.9281, 75) centre (7.9281, 85) ccw
  line L101 (-2.0719, 85) -> (-2.0719, 100)
  arc A46 (7.9281, 110) -> (-2.0719, 100) centre (7.9281, 100) ccw
  line L102 (7.9281, 110) -> (12.9316, 110)
  arc A47 (22.9316, 100) -> (12.9316, 110) centre (12.9316, 100) ccw
  line L103 (-40, 30) -> (-110, 30)
  arc A48 (-120, 40) -> (-110, 30) centre (-110, 40) ccw
  line L104 (-120, 40) -> (-120, 60)
  arc A49 (-110, 70) -> (-120, 60) centre (-110, 60) ccw
  line L105 (-110, 70) -> (-40, 70)
  arc A50 (-30, 60) -> (-40, 70) centre (-40, 60) ccw
  line L106 (-30, 60) -> (-30, 40)
  arc A51 (-40, 30) -> (-30, 40) centre (-40, 40) ccw
  line L107 (-10, 70) -> (10, 70)
  arc A52 (20, 60) -> (10, 70) centre (10, 60) ccw
  line L108 (20, 60) -> (20, 40)
  arc A53 (10, 30) -> (20, 40) centre (10, 40) ccw
  line L109 (10, 30) -> (-10, 30)
  arc A54 (-20, 40) -> (-10, 30) centre (-10, 40) ccw
  line L110 (-20, 40) -> (-20, 60)
  arc A55 (-10, 70) -> (-20, 60) centre (-10, 60) ccw
  ellipse E0 centre (22.741, -39.3535) end of major axis (22.741, -46.5838) minor radius 7 (22.741, -46.5838) -> (29.741, -39.3535) ccw
  line L111 (29.741, -39.3535) -> (29.741, 209.5755)
  ellipse E1 centre (22.741, 209.5755) end of major axis (22.741, 216.8058) minor radius 7 (29.741, 209.5755) -> (22.741, 216.8058) ccw
  line L112 (22.741, 216.8058) -> (-123.259, 216.8058)
  ellipse E2 centre (-123.259, 209.5755) end of major axis (-123.259, 216.8058) minor radius 7 (-123.259, 216.8058) -> (-130.259, 209.5755) ccw
  line L113 (-130.259, 209.5755) -> (-130.259, -39.3535)
  ellipse E3 centre (-123.259, -39.3535) end of major axis (-123.259, -46.5838) minor radius 7 (-130.259, -39.3535) -> (-123.259, -46.5838) ccw
  line L114 (-123.259, -46.5838) -> (22.741, -46.5838)
  line L115 (-35.9419, 179.9959) -> (-35.9419, 150.9959)
  line L116 (-35.9419, 150.9959) -> (-72.9419, 150.9959)
  line L117 (-72.9419, 150.9959) -> (-72.9419, 179.9959)
  line L118 (-72.9419, 179.9959) -> (-35.9419, 179.9959)
  line L119 (-60.0369, -37.2933) -> (-30, -37.2933)
  line L120 (-30, -37.2933) -> (-30, -55)
  line L121 (-30, -55) -> (-60.0369, -55)
  line L122 (-60.0369, -55) -> (-60.0369, -37.2933)
  line L123 (-30.1991, 10) -> (-30.1991, -39.3535)
  line L124 (-60, -39.3535) -> (-60, 10)
  line L125 (-60, 10) -> (-30.1991, 10)
  constraint horizontal L119
  constraint vertical L120
  constraint horizontal L121
  constraint vertical L122
move_body "Move7" bodies 1 to x (1, 0, 0) y (0, 1, 0) z (0, 0, 1) at (-233.3232, -32.3399, -120.6943) in component "axe"
sketch "Sketch72" plane through (30.1991, 0, 0) normal (1, 0, 0) x (0, 0, -1)
  line L0 (66.3857, 103.6645) -> (67.1622, 106.5623)
  line L1 (21.4803, 118.8027) -> (20.7039, 115.9049)
  line L2 (20.7039, 115.9049) -> (66.3857, 103.6645)
  line L3 (21.4803, 118.8027) -> (67.1622, 106.5623)
  line L4 (66.3857, 103.6645) -> (67.1622, 106.5623)
  line L5 (66.3857, 103.6645) -> (20.7039, 115.9049)
  line L6 (20.7039, 115.9049) -> (21.4803, 118.8027)
  line L7 (67.1622, 106.5623) -> (21.4803, 118.8027)
  constraint coincident L1.start L3.start
  constraint coincident L0.end L3.end
  constraint coincident L0.start L2.end
  constraint coincident L1.end L2.start
sketch "Sketch73" plane through (60, 0, 0) normal (-1, 0, 0) x (0, 0, 1)
  line L0 (-67.1622, 106.5623) -> (-66.3857, 103.6645)
  line L1 (-66.3857, 103.6645) -> (-20.7039, 115.9049)
  line L2 (-20.7039, 115.9049) -> (-21.4803, 118.8027)
  line L3 (-21.4803, 118.8027) -> (-66.7739, 105.1134)
  line L4 (-66.7739, 105.1134) -> (-66.3857, 103.6645)
  line L5 (-66.3857, 103.6645) -> (-20.7039, 115.9049)
  line L6 (-21.4803, 118.8027) -> (-20.7039, 115.9049)
  line L7 (-21.4803, 118.8027) -> (-67.1622, 106.5623)
  constraint coincident L2.end L3.start
  constraint midpoint L0 L3.end
  constraint coincident L0.end L1.start
  constraint coincident L1.end L2.start
sketch "Sketch74" plane through (0, 113.3167, -30.3631) normal (0, -0.965926, 0.258819) x (1, 0, 0)
  line L0 (30, -37.2933) -> (36.1991, -37.2933)
  line L1 (36.1991, -37.2933) -> (36.1991, 10)
  line L2 (36.1991, 10) -> (60, 10)
  line L3 (60.0369, -37.2933) -> (60.0369, -44.2609)
  line L4 (60.0369, -44.2609) -> (127.259, -44.2609)
  line L5 (127.259, -44.2609) -> (127.259, 212.9313)
  line L6 (127.259, 212.9313) -> (-26.741, 212.9313)
  line L7 (-26.741, 212.9313) -> (-26.741, -44.2609)
  line L8 (-26.741, -44.2609) -> (30, -44.2609)
  line L9 (30, -44.2609) -> (30, -37.2933)
  line L10 (35.9419, 150.9959) -> (35.9419, 179.9959)
  line L11 (35.9419, 179.9959) -> (72.9419, 179.9959)
  line L12 (72.9419, 179.9959) -> (72.9419, 150.9959)
  line L13 (72.9419, 150.9959) -> (35.9419, 150.9959)
  line L14 (31.3901, -25) -> (16.3901, -25)
  line L15 (16.3901, -25) -> (16.3901, 5)
  line L16 (16.3901, 5) -> (31.3901, 5)
  line L17 (31.3901, 5) -> (31.3901, -25)
  line L18 (60, 10) -> (60, -37.2933)
  line L19 (60, -37.2933) -> (60.0369, -37.2933)
  dimension "d284" = 15
  dimension "d285" = 30
  constraint horizontal L14
  constraint vertical L15
  constraint horizontal L16
  constraint vertical L17
  measures "d284" distance of L14.start L14.end
  measures "d285" distance of L14.start L16.end
move_body "Move8" bodies 1 to x (1, 0, 0) y (0, 1, 0) z (0, 0, 1) at (0, 18.0244, -10.006) in component "axe"
sketch "Sketch75" plane through (39.0666, 0, 0) normal (-1, 0, 0) x (0, 0, 1)
  line L0 (-43.5599, 98.1845) -> (-25.4349, 103.0411)
  line L1 (-25.4349, 103.0411) -> (-54.2221, 210.4766)
  line L2 (-54.2221, 210.4766) -> (-35.2373, 215.5636)
  line L3 (-35.2373, 215.5636) -> (-36.9436, 221.9319)
  line L4 (-49.1911, 229.0029) -> (-94.7668, 216.791)
  line L5 (-94.7668, 216.791) -> (-90.4722, 200.7634)
  line L6 (-90.4722, 200.7634) -> (-72.3472, 205.62)
  line L7 (-72.3472, 205.62) -> (-43.5599, 98.1845)
  circle A0 centre (-37, 106) radius 2.5
  arc A1 (-36.9436, 221.9319) -> (-49.1911, 229.0029) centre (-46.6029, 219.3437) ccw
  dimension "d288" = 5
  measures "d288" diameter of A0
extrude "Extrude2" cut sketch "Sketch75" against normal blind 15 contours A0 in component "axe"
move_body "Move9" bodies 1 to x (1, 0, 0) y (0, 0.996195, 0.087156) z (0, -0.087156, 0.996195) at (0, -3.4229, -8.7231) in component "axe"